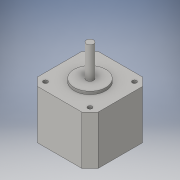
# Autodesk Inventor part: NEMA16 Motor
Saved by Autodesk Inventor 2016 (Build 200138000, 138)
## iProperties
Created: 2016-04-25
Part Number: NEMA16 Motor
Material: Generic
Document SubType Name: Modeling
Designer: rubenjm
Density: 1 g/cm^3
Appearance: Default
Author: rubenjm
Autodesk Inventor part; units mm, degrees
ref_plane "YZ Plane" through (0, 0, 0) normal (1, 0, 0) x (0, 1, 0)
ref_plane "XZ Plane" through (0, 0, 0) normal (0, 1, 0) x (-1, 0, 0)
ref_plane "XY Plane" through (0, 0, 0) normal (0, 0, 1) x (1, 0, 0)
sketch "Sketch1" plane through (0, 0, 0) normal (0, 1, 0) x (-1, 0, 0)
  line L0 (0, -5.65) -> (0, -36.65)
  line L1 (36.65, -42.3) -> (5.65, -42.3)
  line L2 (42.3, -36.65) -> (42.3, -5.65)
  line L3 (5.65, 0) -> (36.65, 0)
  line L4 (36.65, 0) -> (42.3, -5.65)
  line L5 (42.3, -36.65) -> (36.65, -42.3)
  line L6 (5.65, -42.3) -> (0, -36.65)
  line L7 (0, -5.65) -> (5.65, 0)
  line L8 (5.65, -36.65) -> (36.65, -36.65) construction
  line L9 (36.65, -36.65) -> (36.65, -5.65) construction
  line L10 (36.65, -5.65) -> (5.65, -5.65) construction
  line L11 (5.65, -5.65) -> (5.65, -36.65) construction
  line L12 (5.65, -36.65) -> (36.65, -5.65) construction
  line L13 (36.65, -36.65) -> (5.65, -5.65) construction
  circle A0 centre (36.65, -5.65) radius 1.5
  circle A1 centre (36.65, -36.65) radius 1.5
  circle A2 centre (5.65, -36.65) radius 1.5
  circle A3 centre (5.65, -5.65) radius 1.5
  point P0 (0, 0)
  point P1 (21.15, -21.15)
  dimension "d12" = 3
  dimension "d14" = 3
  dimension "d15" = 3
  constraints: 28 end point, 4 centre point, 2 midpoint, 2 parallel, 2 perpendicular, 1 coincident, 1 horizontal
  measures "d12" diameter of A0
  measures "d14" diameter of A2
  measures "d15" diameter of A3
extrude "Extrusion1" add sketch "Sketch1" along normal blind 34
sketch "Sketch2" plane through (0, 34, 0) normal (0, 1, 0) x (1, 0, 0)
  line L0 (-42.3, 5.65) -> (-36.65, 0) construction
  line L1 (-39.475, 2.825) -> (-2.825, 39.475) construction
  line L2 (0, 36.65) -> (-5.65, 42.3) construction
  line L3 (-36.65, 42.3) -> (-42.3, 36.65) construction
  line L4 (-39.475, 39.475) -> (-2.825, 2.825) construction
  line L5 (-5.65, 0) -> (0, 5.65) construction
  circle A0 centre (-21.15, 21.15) radius 11
  point P0 (0, 0)
  dimension "d18" = 22
  constraints: 5 midpoint, 4 end point, 1 centre point
  measures "d18" diameter of A0
extrude "Extrusion2" add sketch "Sketch2" along normal blind 2
sketch "Sketch3" plane through (-21.15, 36, -21.15) normal (0, 1, 0) x (1, 0, 0)
  line L0 (-21.15, -15.5) -> (-15.5, -21.15) construction
  line L1 (-18.325, -18.325) -> (18.325, 18.325) construction
  line L2 (21.15, 15.5) -> (15.5, 21.15) construction
  line L3 (-18.325, 18.325) -> (18.325, -18.325) construction
  line L4 (15.5, -21.15) -> (21.15, -15.5) construction
  circle A0 centre (0, 0) radius 2.5
  point P0 (21.15, -21.15)
  dimension "d21" = 5
  constraints: 4 end point, 4 midpoint, 1 centre point
  measures "d21" diameter of A0
extrude "Extrusion3" add sketch "Sketch3" along normal blind 22
body "Solid1"
